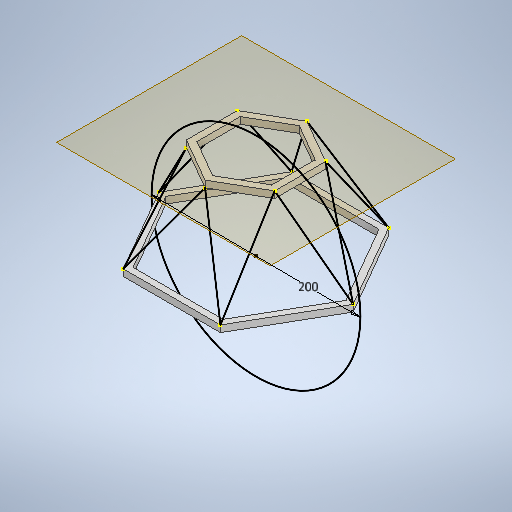
# Autodesk Inventor part: Straight Dome
Saved by Autodesk Inventor 2025.1 (Build 291241000, 241)
## iProperties
Created: 2024-11-11
Part Number: Straight Dome
Material: Generic
Document SubType Name: Modeling
Designer: monos
Density: 1 g/cm^3
Appearance: Default
Author: monos
Autodesk Inventor part; units mm, degrees
ref_plane "YZ Plane" through (0, 0, 0) normal (1, 0, 0) x (0, 1, 0)
ref_plane "XY Plane" through (0, 0, 0) normal (0, 0, 1) x (1, 0, 0)
sketch "Sketch1" plane through (0, 0, 0) normal (0, 1, 0) x (-1, 0, 0)
  line L0 (93, 0) -> (46.5, -80.5404)
  line L1 (46.5, -80.5404) -> (-46.5, -80.5404)
  line L2 (-46.5, -80.5404) -> (-93, 0)
  line L3 (-93, 0) -> (-46.5, 80.5404)
  line L4 (-46.5, 80.5404) -> (46.5, 80.5404)
  line L5 (46.5, 80.5404) -> (93, 0)
  line L6 (43.0992, -74.65) -> (-43.0992, -74.65)
  line L7 (-43.0992, -74.65) -> (-86.1984, 0)
  line L8 (-86.1984, 0) -> (-43.0992, 74.65)
  line L9 (-43.0992, 74.65) -> (43.0992, 74.65)
  line L10 (43.0992, 74.65) -> (86.1984, 0)
  line L11 (86.1984, 0) -> (43.0992, -74.65)
  point P0 (0, 0)
  point P1 (0, 0)
  point P2 (0, 0)
  constraints: 24 end point, 26 other
extrude "Extrusion1" add sketch "Sketch1" along normal blind 6.35
ref_plane "Work Plane1" through (0, 87.3, 0) normal (0, 1, 0) x (-1, 0, 0)
sketch "Sketch2" plane through (0, 0, 0) normal (0, 0, 1) x (1, 0, 0)
  circle A0 centre (0, 0) radius 100
  dimension "d5" = 200
  constraints: 1 centre point, 1 coincident
  measures "d5" diameter of A0
sketch "Sketch3" plane through (0, 87.3, 0) normal (0, 1, 0) x (-1, 0, 0)
  line L0 (-86.1984, 0) -> (-43.0992, 74.65) projected
  line L1 (-42.2361, 24.385) -> (0, 48.77)
  line L2 (0, 48.77) -> (42.2361, 24.385)
  line L3 (42.2361, 24.385) -> (42.2361, -24.385)
  line L4 (42.2361, -24.385) -> (0, -48.77)
  line L5 (0, -48.77) -> (-42.2361, -24.385)
  line L6 (-42.2361, -24.385) -> (-42.2361, 24.385)
  line L7 (0, 41.4376) -> (35.886, 20.7188)
  line L8 (35.886, 20.7188) -> (35.886, -20.7188)
  line L9 (35.886, -20.7188) -> (0, -41.4376)
  line L10 (0, -41.4376) -> (-35.886, -20.7188)
  line L11 (-35.886, -20.7188) -> (-35.886, 20.7188)
  line L12 (-35.886, 20.7188) -> (0, 41.4376)
  point P0 (0, 0)
  constraints: 24 end point, 13 other
extrude "Extrusion2" add sketch "Sketch3" against normal blind 6.35
sketch3d "3D Sketch1"
body "Solid1"
